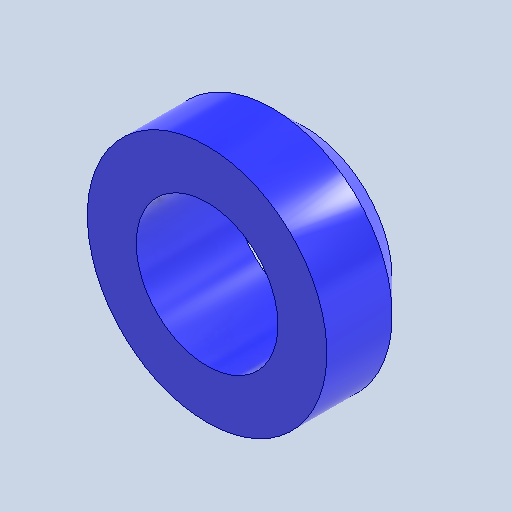
# Autodesk Inventor part: roja-v1-3DP-rotate-spesa
Saved by Autodesk Inventor 2025.2 (Build 292293000, 293)
## iProperties
Created: 2024-08-05
Part Number: roja-v1-3DP-rotate-spesa
Material: ABS プラスチック
Document SubType Name: Modeling
Designer: haruy
Density: 1.06 g/cm^3
Appearance: 青 - 壁塗料 - 光沢
Author: haruy
Autodesk Inventor part; units mm, degrees
ref_plane "YZ Plane" through (0, 0, 0) normal (1, 0, 0) x (0, 1, 0)
ref_plane "XZ Plane" through (0, 0, 0) normal (0, 1, 0) x (-1, 0, 0)
ref_plane "XY Plane" through (0, 0, 0) normal (0, 0, 1) x (1, 0, 0)
sketch "スケッチ1" plane through (0, 0, 0) normal (1, 0, 0) x (0, 1, 0)
  line L0 (4.6242, 11.445) -> (4.6242, -2.555)
  line L1 (11.6242, 11.445) -> (11.6242, 2.095)
  line L2 (4.6242, -2.555) -> (6.9742, -2.555)
  line L3 (6.9742, -2.555) -> (6.9742, -0.555) construction
  line L4 (6.9742, -0.555) -> (4.6242, -0.555) construction
  line L5 (4.6242, -0.555) -> (4.6242, -2.555)
  line L6 (6.9742, -0.555) -> (13.5918, -0.555) construction
  line L7 (6.9742, -2.555) -> (11.6242, 2.095)
  line L8 (6.9742, -2.555) -> (13.5503, -2.555) construction
  line L9 (11.6242, 11.445) -> (4.6242, 11.445)
  line L10 (4.6242, 11.445) -> (11.4742, 11.445)
  line L11 (11.4742, 11.445) -> (11.4742, 4.445)
  line L12 (11.4742, 4.445) -> (4.6242, 4.445)
  line L13 (4.6242, 4.445) -> (4.6242, 11.445)
  line L14 (-5.5258, -6.545) -> (-5.5258, 15.435)
  line L15 (11.4742, 4.445) -> (11.6242, 4.595)
  point P0 (0, 0)
  point P1 (-5.5258, 4.445)
  point P2 (4.6242, 4.445)
  point P3 (11.6242, 6.77)
  point P4 (11.7242, 5.295)
  point P5 (11.4742, 12.295)
  point P6 (4.7242, 5.295)
  dimension "d0" = 10.15
  dimension "d1" = 7
  dimension "d2" = 14
  dimension "d3" = 2
  dimension "d4" = 12.5
  dimension "d5" = 45
  dimension "d6" = 7
  dimension "d7" = 17
  dimension "d8" = 45
  constraints: 32 end point, 4 horizontal, 4 parallel, 3 perpendicular, 2 horizontal alignment, 2 midpoint, 1 equal length, 1 point on line, 1 vertical
  measures "d0" distance from line of point (-5.526, 4.445) L0
  measures "d1" distance between parallel lines of L0 L1
  measures "d2" distance of L0.start L0.end
  measures "d3" distance between parallel lines of L2 L4
  measures "d4" distance from line of point (-5.526, 4.445) L3
  measures "d5" angle of L8 L7
  measures "d6" distance of L10.end L11.end
  measures "d7" horizontal distance of point (-5.526, 4.445) L10.end
  measures "d8" angle of L15 L11
revolve "回転1" add sketch "スケッチ1" angle 360 about axis through (0, -5.5258, -6.545) along (0, 0, 1)
